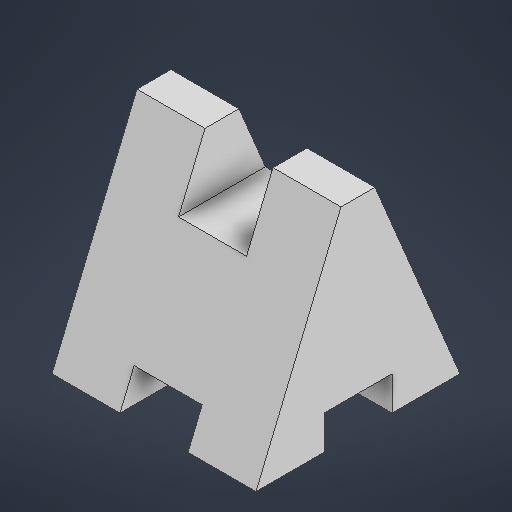
# Autodesk Inventor part: b4
Saved by Autodesk Inventor 2025.4 (Build 294407000, 407)
## iProperties
Created: 2026-05-07
Part Number: b4
Material: Generic
Document SubType Name: Modeling
Designer: VuQuan
Density: 1 g/cm^3
Appearance: Default
Author: VuQuan
Autodesk Inventor part; units mm, degrees
ref_plane "YZ Plane" through (0, 0, 0) normal (1, 0, 0) x (0, 1, 0)
ref_plane "XZ Plane" through (0, 0, 0) normal (0, 1, 0) x (-1, 0, 0)
ref_plane "XY Plane" through (0, 0, 0) normal (0, 0, 1) x (1, 0, 0)
sketch "Sketch1" plane through (0, 0, 0) normal (0, 0, 1) x (1, 0, 0)
  line L0 (0, 0) -> (15, 0)
  line L1 (15, 0) -> (15, -15)
  line L2 (15, -15) -> (45, -15)
  line L3 (45, -15) -> (45, 75)
  line L4 (45, 75) -> (15, 75)
  line L5 (15, 75) -> (15, 47)
  line L6 (15, 47) -> (0, 47)
  line L7 (0, 0) -> (0, 47) construction
  line L8 (0, 0) -> (-15, 0)
  line L9 (-15, 0) -> (-15, -15)
  line L10 (-15, -15) -> (-45, -15)
  line L11 (-45, -15) -> (-45, 75)
  line L12 (-45, 75) -> (-15, 75)
  line L13 (-15, 75) -> (-15, 47)
  line L14 (-15, 47) -> (0, 47)
  dimension "d0" = 47
  dimension "d1" = 28
  dimension "d2" = 30
  dimension "d3" = 15
  dimension "d4" = 90
  constraints: 30 end point, 6 symmetric about line, 4 perpendicular, 4 point on line, 1 horizontal, 1 vertical, 1 vertical alignment
  measures "d0" distance between parallel lines of L0 L6
  measures "d1" distance between parallel lines of L4 L6
  measures "d2" distance of L1.end L2.end
  measures "d3" distance of L0.end L1.end
  measures "d4" distance between parallel lines of L3 L11
extrude "Extrusion1" add sketch "Sketch1" along normal blind 90
sketch "Sketch2" plane through (-45, -15, 0) normal (-1, 0, 0) x (0, 0, 1)
  line L0 (0, 90) -> (0, 0) projected
  line L1 (0, 0) -> (90, 0) projected
  line L2 (90, 90) -> (90, 0) projected
  line L3 (0, 90) -> (90, 90) projected
  line L4 (90, 15) -> (90, 0) projected
  line L5 (90, 0) -> (52.5, 90)
  line L6 (0, 90) -> (90, 90) projected
  line L7 (37.5, 90) -> (0, 0)
  line L8 (30, 0) -> (30, 15)
  line L9 (30, 15) -> (60, 15)
  line L10 (60, 15) -> (60, 0)
  point P0 (0, 15)
  point P1 (45, 15)
  point P2 (45, 0)
  dimension "d12" = 30
  dimension "d13" = 15
  constraints: 10 end point, 5 point on line, 2 midpoint, 2 perpendicular, 1 equal length, 1 vertical, 1 vertical alignment
  measures "d12" distance of L8.end L9.end
  measures "d13" distance of L5.end L7.start
extrude "Extrusion2" cut sketch "Sketch2" against normal blind 90 contours L3 L7 L0 | L8 L9 L10 L1 | L3 L2 L5
body "Solid1"
